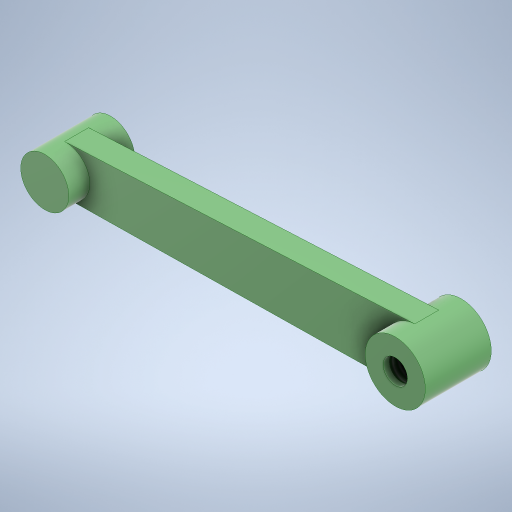
# Autodesk Inventor part: DualPMTController.ScreenSpacer
Saved by Autodesk Inventor 2023 (Build 270158000, 158)
## iProperties
Created: 2023-09-26
Part Number: DualPMTController.ScreenSpacer
Material: Generic
Document SubType Name: Modeling
Designer: Graeme
Density: 1 g/cm^3
Appearance: Default
Author: Graeme
Autodesk Inventor part; units mm, degrees
ref_plane "YZ Plane" through (0, 0, 0) normal (1, 0, 0) x (0, 1, 0)
sketch "Sketch4" plane through (0, 0, 0) normal (0, 0, 1) x (1, 0, 0)
  circle A0 centre (49.58, 12.36) radius 1.25 projected
  circle A1 centre (49.58, -8.84) radius 1.25 projected
  line L0 (43.38, -11.54) -> (43.38, 15.06) projected
  line L1 (43.38, 15.06) -> (16.78, 15.06) projected
  line L2 (16.78, 15.06) -> (16.78, -11.54) projected
  line L3 (16.78, -11.54) -> (43.38, -11.54) projected
  line L4 (41.7543, -9.9143) -> (18.4057, -9.9143) projected
  line L5 (18.4057, -9.9143) -> (18.4057, 13.4343) projected
  line L6 (18.4057, 13.4343) -> (41.7543, 13.4343) projected
  line L7 (41.7543, 13.4343) -> (41.7543, -9.9143) projected
  circle A2 centre (20.4057, 11.4343) radius 2
  circle A3 centre (49.58, 12.36) radius 2.5
  point P0 (0, 0)
  dimension "d8" = 4
  dimension "d9" = 5
  constraints: 2 centre point, 2 tangent, 1 coincident
  measures "d8" diameter of A2
  measures "d9" diameter of A3
ref_plane "Work Plane3" through (16.78, -11.54, 5.4873) normal (0, 0, -1) x (0, 1, 0)
extrude "Extrusion3" add sketch "Sketch4" along normal up to surface (5.4873 mm away) contours A0 | A2 | A3
ref_plane "Work Plane4" through (20.4057, 11.4343, 2.7437) normal (0, 0, 1) x (1, 0, 0)
sketch "Sketch5" plane through (20.4057, 11.4343, 2.7437) normal (0, 0, 1) x (1, 0, 0)
  circle A0 centre (0, 0) radius 2 projected
  circle A1 centre (29.1743, 0.9257) radius 2.5 projected
  line L0 (-0.0977, 1.9976) -> (29.0523, 3.4227)
  circle A2 centre (29.1743, 0.9257) radius 2.5 projected
  line L1 (29.2108, -1.5741) -> (0.0292, -1.9998)
  point P0 (-20.4057, -11.4343)
  point P1 (29.0523, 3.4227)
  constraints: 4 end point, 2 point on circle, 2 tangent, 6 other
extrude "Extrusion4" add sketch "Sketch5" along normal mid plane 2 contours A0 L0 A1 L1
sketch "Sketch6" plane through (49.58, 12.36, 0) normal (0, 0, -1) x (-1, 0, 0)
  circle A0 centre (0, 0) radius 2.5 projected
  point P0 (49.58, -12.36)
  constraints: 1 coincident
hole "Hole1" at (49.58, 12.36, 0) direction (0, 0, 1) diameter 2.013 end through all thread size "M2.5x0.45" class "6H" standard "ISO Metric profile"
body "Solid2"
